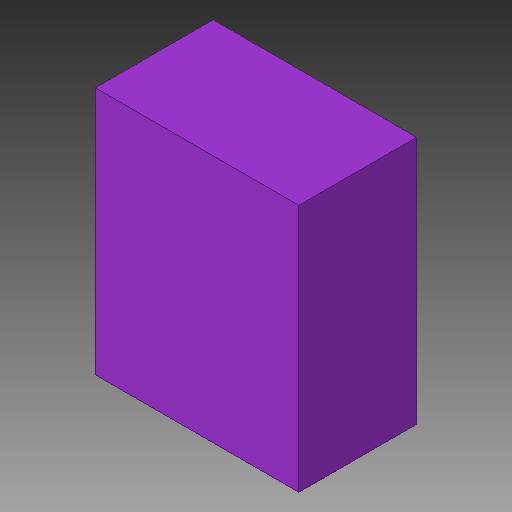
# Autodesk Inventor part: TPS62237DRY
Saved by Autodesk Inventor 2018 (Build 220112000, 112)
## iProperties
Created: 2015-11-24
Part Number: TPS62237DRY
Material: Generic
Document SubType Name: Modeling
Designer: PhillipD
Density: 1 g/cm^3
Appearance: DRY6, TPS62237DRY
Author: PhillipD
Autodesk Inventor part; units mm, degrees
ref_plane "YZ Plane" through (0, 0, 0) normal (1, 0, 0) x (0, 1, 0)
ref_plane "XZ Plane" through (0, 0, 0) normal (0, 1, 0) x (-1, 0, 0)
ref_plane "XY Plane" through (0, 0, 0) normal (0, 0, 1) x (1, 0, 0)
sketch "DRY6, TPS62237DRY_173" plane through (0, 0, 0) normal (0, 0, 1) x (1, 0, 0)
  line L0 (-0.8636, 1.016) -> (0.8636, 1.016)
  line L1 (0.8636, 1.016) -> (0.8636, -1.0922)
  line L2 (0.8636, -1.0922) -> (-0.8636, -1.0922)
  line L3 (-0.8636, -1.0922) -> (-0.8636, 1.016)
  constraints: 8 end point
extrude "Extrusion1" add sketch "DRY6, TPS62237DRY_173" along normal blind 1
body "Solid1"
